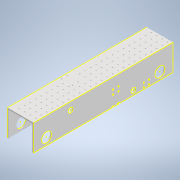
# Autodesk Inventor part: Side Channel
Saved by Autodesk Inventor 2021 (Build 250183000, 183)
## iProperties
Created: 2019-12-09
Part Number: Side Channel
Material: Generic
Document SubType Name: Modeling
Designer: deli
Density: 1 g/cm^3
Appearance: Default
Author: deli
Autodesk Inventor part; units mm, degrees
ref_plane "YZ Plane" through (0, 0, 0) normal (1, 0, 0) x (0, 1, 0)
ref_plane "XZ Plane" through (0, 0, 0) normal (0, 1, 0) x (-1, 0, 0)
ref_plane "XY Plane" through (0, 0, 0) normal (0, 0, 1) x (1, 0, 0)
sketch "Sketch1" plane through (0, 0, 0) normal (0, 0, 1) x (1, 0, 0)
  line L0 (-186.621, 45.7633) -> (-110.421, 45.7633)
  line L1 (-110.421, 45.7633) -> (-110.421, -30.4367)
  line L2 (-110.421, -30.4367) -> (-186.621, -30.4367)
  line L3 (-186.621, -30.4367) -> (-186.621, 45.7633)
  line L4 (-183.446, 42.5883) -> (-113.596, 42.5883)
  line L5 (-113.596, 42.5883) -> (-113.596, -27.2617)
  line L6 (-113.596, -27.2617) -> (-183.446, -27.2617)
  line L7 (-183.446, -27.2617) -> (-183.446, 42.5883)
  point P0 (0, 0)
  dimension "d0" = 76.2
  dimension "d1" = 76.2
  dimension "d2" = 3.175
  dimension "d3" = 3.175
  dimension "d4" = 3.175
  dimension "d5" = 3.175
  constraints: 16 end point, 4 parallel, 2 horizontal, 2 perpendicular
  measures "d0" distance of L1.end L2.end
  measures "d1" distance of L0.end L1.end
  measures "d2" distance between parallel lines of L0 L4
  measures "d3" distance between parallel lines of L1 L5
  measures "d4" distance between parallel lines of L2 L6
  measures "d5" distance between parallel lines of L3 L7
extrude "Extrusion1" add sketch "Sketch1" along normal blind 406.4
sketch "Sketch2" plane through (0, 0, 406.4) normal (0, 0, 1) x (1, 0, 0)
  line L0 (-113.596, 42.5883) -> (-113.596, -27.2617) projected
  line L1 (-183.446, -27.2617) -> (-183.446, 42.5883) projected
  line L2 (-186.621, -30.4367) -> (-110.421, -30.4367) projected
  line L3 (-183.446, -27.2617) -> (-113.596, -27.2617)
  line L4 (-113.596, -27.2617) -> (-113.596, -30.4367)
  line L5 (-113.596, -30.4367) -> (-183.446, -30.4367)
  line L6 (-183.446, -30.4367) -> (-183.446, -27.2617)
  point P0 (0, 0)
  constraints: 8 end point, 2 parallel, 1 horizontal, 1 perpendicular, 1 point on line
extrude "Extrusion2" cut sketch "Sketch2" against normal blind 457.2
sketch "Sketch3" plane through (-110.421, -30.4367, 0) normal (1, 0, 0) x (0, 0, -1)
  circle A0 centre (-368.3, 20.8534) radius 14.5034
  line L0 (-406.4, 0) -> (-406.4, 76.2) projected
  line L1 (0, 0) -> (-406.4, 0) projected
  circle A1 centre (-38.1, 20.8534) radius 14.5034
  line L2 (0, 0) -> (0, 76.2) projected
  point P0 (0, 30.4367)
  dimension "d10" = 29.0068
  dimension "d11" = 38.1
  dimension "d12" = 20.8534
  dimension "d13" = 29.0068
  dimension "d14" = 38.1
  dimension "d15" = 20.8534
  constraints: 2 centre point
  measures "d10" diameter of A0
  measures "d11" distance from line of A0.centre L0
  measures "d12" distance from line of L1 A0.centre
  measures "d13" diameter of A1
  measures "d14" distance from line of L2 A1.centre
  measures "d15" distance from line of L1 A1.centre
extrude "Extrusion3" cut sketch "Sketch3" against normal blind 76.2
sketch "Sketch4" plane through (-186.621, -30.4367, 0) normal (-1, 0, 0) x (0, 0, 1)
  circle A0 centre (115.1699, 12.7) radius 6.9977
  line L0 (0, 76.2) -> (406.4, 76.2) projected
  circle A1 centre (38.1, 20.8534) radius 14.5034 projected
  circle A2 centre (38.1, 20.8534) radius 50.8
  line L1 (0, 0) -> (406.4, 0) projected
  line L2 (88.9, 0) -> (88.9, 76.2)
  circle A3 centre (298.2343, 53.975) radius 6.9977
  circle A4 centre (368.3, 20.8534) radius 2.55 projected
  point P0 (0, 30.4367)
  dimension "d18" = 13.9954
  dimension "d20" = 101.6
  dimension "d21" = 77.5
  dimension "d24" = 13.9954
  dimension "d25" = 22.225
  dimension "d26" = 77.5
  dimension "d31" = 12.7
  constraints: 3 centre point, 2 end point, 2 point on line, 1 coincident, 1 perpendicular
  measures "d18" diameter of A0
  measures "d20" diameter of A2
  measures "d21" distance of A0.centre A2.centre
  measures "d24" diameter of A3
  measures "d25" distance from line of L0 A3.centre
  measures "d26" distance of A3.centre A4.centre
  measures "d31" distance from line of L1 A0.centre
extrude "Extrusion5" cut sketch "Sketch4" against normal blind 127 contours A0 | A3
sketch "Sketch5" plane through (-186.621, 45.7633, 0) normal (0, 1, 0) x (1, 0, 0)
  circle A0 centre (6.225, -254.5181) radius 1.8542
  circle A1 centre (6.225, -238.5181) radius 1.8542
  circle A2 centre (38.225, -238.5181) radius 1.8542
  circle A3 centre (38.225, -254.5181) radius 1.8542
  circle A4 centre (6.225, -254.5181) radius 2.8702 projected
  circle A5 centre (38.225, -254.5181) radius 2.5146 projected
  circle A6 centre (38.225, -238.5181) radius 2.5146 projected
  point P0 (186.621, 0)
  dimension "d36" = 3.7084
  dimension "d37" = 0
  dimension "d38" = 0
  dimension "d39" = 0
  dimension "d40" = 3.7084
  dimension "d41" = 3.7084
  dimension "d42" = 3.7084
  constraints: 4 centre point
  measures "d36" diameter of A1
  measures "d37" distance of A4.centre A0.centre
  measures "d38" distance of A5.centre A3.centre
  measures "d39" distance of A6.centre A2.centre
  measures "d40" diameter of A0
  measures "d41" diameter of A3
  measures "d42" diameter of A2
extrude "Extrusion6" cut sketch "Sketch5" against normal blind 25.4 contours A0 | A1 | A2 | A3
sketch "Sketch6" plane through (-110.421, -30.4367, 0) normal (1, 0, 0) x (0, 0, -1)
  circle A0 centre (-158.8823, 31.875) radius 1.8542
  circle A1 centre (-174.8823, 31.875) radius 1.8542
  circle A2 centre (-174.8823, -0.125) radius 1.8542
  circle A3 centre (-158.8823, -0.125) radius 1.8542
  circle A4 centre (-174.8823, 44.45) radius 1.8542
  circle A5 centre (-158.8823, 44.45) radius 1.8542
  circle A6 centre (-174.8823, -0.125) radius 3.81
  circle A7 centre (-158.8823, -0.125) radius 3.81
  circle A8 centre (-85.09, 17.145) radius 1.8542
  circle A9 centre (-85.09, 5.08) radius 1.8542
  circle A10 centre (-69.85, 5.08) radius 1.8542
  circle A11 centre (-69.85, 17.145) radius 1.8542
  line L0 (0, 0) -> (0, 76.2) projected
  line L1 (0, 0) -> (-406.4, 0) projected
  point P0 (0, 30.4367)
  dimension "d34" = 7.62
  dimension "d35" = 7.62
  dimension "d43" = 3.7084
  dimension "d44" = 3.7084
  dimension "d45" = 3.7084
  dimension "d46" = 3.7084
  dimension "d47" = 3.7084
  dimension "d48" = 3.7084
  dimension "d49" = 11.5316
  dimension "d50" = 15.24
  dimension "d51" = 12.065
  dimension "d52" = 12.065
  dimension "d53" = 15.7292
  dimension "d54" = 69.85
  dimension "d55" = 3.7084
  dimension "d56" = 3.7084
  dimension "d57" = 3.7084
  dimension "d58" = 3.7084
  dimension "d59" = 5.08
  constraints: 12 centre point, 2 coincident
  measures "d34" diameter of A6
  measures "d35" diameter of A7
  measures "d43" diameter of A5
  measures "d44" diameter of A0
  measures "d45" diameter of A1
  measures "d46" diameter of A4
  measures "d47" diameter of A2
  measures "d48" diameter of A3
  measures "d50" distance of A9.centre A10.centre
  measures "d51" distance of A11.centre A10.centre
  measures "d52" distance of A8.centre A9.centre
  measures "d54" distance from line of L0 A11.centre
  measures "d55" diameter of A11
  measures "d56" diameter of A8
  measures "d57" diameter of A9
  measures "d58" diameter of A10
  measures "d59" distance from line of L1 A10.centre
extrude "Extrusion7" cut sketch "Sketch6" against normal blind 25.4
sketch "Sketch7" plane through (-186.621, 45.7633, 0) normal (0, 1, 0) x (1, 0, 0)
  circle A0 centre (20.2, -7.62) radius 1.65
  circle A1 centre (38.225, -254.5181) radius 1.8542 projected
  circle A2 centre (6.225, -238.5181) radius 1.8542 projected
  circle A3 centre (38.225, -238.5181) radius 1.8542 projected
  circle A4 centre (6.225, -254.5181) radius 1.8542 projected
  line L0 (76.2, 0) -> (0, 0) projected
  line L1 (0, 0) -> (0, -406.4) projected
  line L2 (76.2, -406.4) -> (0, -406.4) projected
  line L3 (76.2, 0) -> (76.2, -406.4) projected
  circle A5 centre (36.2, -7.62) radius 1.65
  circle A6 centre (52.2, -7.62) radius 1.65
  circle A7 centre (68.2, -7.62) radius 1.65
  circle A8 centre (20.2, -23.62) radius 1.65
  circle A9 centre (36.2, -23.62) radius 1.65
  circle A10 centre (52.2, -23.62) radius 1.65
  circle A11 centre (68.2, -23.62) radius 1.65
  circle A12 centre (20.2, -39.62) radius 1.65
  circle A13 centre (36.2, -39.62) radius 1.65
  circle A14 centre (52.2, -39.62) radius 1.65
  circle A15 centre (68.2, -39.62) radius 1.65
  circle A16 centre (20.2, -55.62) radius 1.65
  circle A17 centre (36.2, -55.62) radius 1.65
  circle A18 centre (52.2, -55.62) radius 1.65
  circle A19 centre (68.2, -55.62) radius 1.65
  circle A20 centre (20.2, -71.62) radius 1.65
  circle A21 centre (36.2, -71.62) radius 1.65
  circle A22 centre (52.2, -71.62) radius 1.65
  circle A23 centre (68.2, -71.62) radius 1.65
  circle A24 centre (20.2, -87.62) radius 1.65
  circle A25 centre (36.2, -87.62) radius 1.65
  circle A26 centre (52.2, -87.62) radius 1.65
  circle A27 centre (68.2, -87.62) radius 1.65
  circle A28 centre (20.2, -103.62) radius 1.65
  circle A29 centre (36.2, -103.62) radius 1.65
  circle A30 centre (52.2, -103.62) radius 1.65
  circle A31 centre (68.2, -103.62) radius 1.65
  circle A32 centre (20.2, -119.62) radius 1.65
  circle A33 centre (36.2, -119.62) radius 1.65
  circle A34 centre (52.2, -119.62) radius 1.65
  circle A35 centre (68.2, -119.62) radius 1.65
  circle A36 centre (20.2, -135.6199) radius 1.65
  circle A37 centre (36.2, -135.6199) radius 1.65
  circle A38 centre (52.2, -135.6199) radius 1.65
  circle A39 centre (68.2, -135.6199) radius 1.65
  circle A40 centre (20.2, -151.6199) radius 1.65
  circle A41 centre (36.2, -151.6199) radius 1.65
  circle A42 centre (52.2, -151.6199) radius 1.65
  circle A43 centre (68.2, -151.6199) radius 1.65
  circle A44 centre (20.2, -167.6199) radius 1.65
  circle A45 centre (36.2, -167.6199) radius 1.65
  circle A46 centre (52.2, -167.6199) radius 1.65
  circle A47 centre (68.2, -167.6199) radius 1.65
  circle A48 centre (20.2, -183.6199) radius 1.65
  circle A49 centre (36.2, -183.6199) radius 1.65
  circle A50 centre (52.2, -183.6199) radius 1.65
  circle A51 centre (68.2, -183.6199) radius 1.65
  circle A52 centre (20.2, -199.6199) radius 1.65
  circle A53 centre (36.2, -199.6199) radius 1.65
  circle A54 centre (52.2, -199.6199) radius 1.65
  circle A55 centre (68.2, -199.6199) radius 1.65
  circle A56 centre (20.2, -215.6199) radius 1.65
  circle A57 centre (36.2, -215.6199) radius 1.65
  circle A58 centre (52.2, -215.6199) radius 1.65
  circle A59 centre (68.2, -215.6199) radius 1.65
  circle A60 centre (20.2, -231.6199) radius 1.65
  circle A61 centre (36.2, -231.6199) radius 1.65
  circle A62 centre (52.2, -231.6199) radius 1.65
  circle A63 centre (68.2, -231.6199) radius 1.65
  circle A64 centre (20.2, -247.6199) radius 1.65
  circle A65 centre (36.2, -247.6199) radius 1.65
  circle A66 centre (52.2, -247.6199) radius 1.65
  circle A67 centre (68.2, -247.6199) radius 1.65
  circle A68 centre (20.2, -263.6199) radius 1.65
  circle A69 centre (36.2, -263.6199) radius 1.65
  circle A70 centre (52.2, -263.6199) radius 1.65
  circle A71 centre (68.2, -263.6199) radius 1.65
  circle A72 centre (20.2, -279.6199) radius 1.65
  circle A73 centre (36.2, -279.6199) radius 1.65
  circle A74 centre (52.2, -279.6199) radius 1.65
  circle A75 centre (68.2, -279.6199) radius 1.65
  circle A76 centre (20.2, -295.6199) radius 1.65
  circle A77 centre (36.2, -295.6199) radius 1.65
  circle A78 centre (52.2, -295.6199) radius 1.65
  circle A79 centre (68.2, -295.6199) radius 1.65
  circle A80 centre (20.2, -311.6199) radius 1.65
  circle A81 centre (36.2, -311.6199) radius 1.65
  circle A82 centre (52.2, -311.6199) radius 1.65
  circle A83 centre (68.2, -311.6199) radius 1.65
  circle A84 centre (20.2, -327.6199) radius 1.65
  circle A85 centre (36.2, -327.6199) radius 1.65
  circle A86 centre (52.2, -327.6199) radius 1.65
  circle A87 centre (68.2, -327.6199) radius 1.65
  circle A88 centre (20.2, -343.6199) radius 1.65
  circle A89 centre (36.2, -343.6199) radius 1.65
  circle A90 centre (52.2, -343.6199) radius 1.65
  circle A91 centre (68.2, -343.6199) radius 1.65
  circle A92 centre (20.2, -359.6199) radius 1.65
  circle A93 centre (36.2, -359.6199) radius 1.65
  circle A94 centre (52.2, -359.6199) radius 1.65
  circle A95 centre (68.2, -359.6199) radius 1.65
  circle A96 centre (20.2, -375.6198) radius 1.65
  circle A97 centre (36.2, -375.6198) radius 1.65
  circle A98 centre (52.2, -375.6198) radius 1.65
  circle A99 centre (68.2, -375.6198) radius 1.65
  circle A100 centre (20.2, -391.6198) radius 1.65
  circle A101 centre (36.2, -391.6198) radius 1.65
  circle A102 centre (52.2, -391.6198) radius 1.65
  circle A103 centre (68.2, -391.6198) radius 1.65
  circle A104 centre (84.2, -71.62) radius 1.65 projected
  circle A105 centre (84.2, -87.62) radius 1.65 projected
  point P0 (186.621, 0)
  dimension "d60" = 3.3
  dimension "d63" = 16
  dimension "d66" = 16
  dimension "d69" = 8
  dimension "d70" = 383.9998
  dimension "d71" = 7.62
  constraints: 100 centre point, 1 horizontal, 1 vertical, 198 other
  measures "d60" diameter of A0
  measures "d63" distance of A0.centre A5.centre
  measures "d66" distance of A0.centre A8.centre
  measures "d69" distance from line of L3 A7.centre
  measures "d70" distance of A102.centre A6.centre
  measures "d71" distance from line of A6.centre L0
extrude "Extrusion8" cut sketch "Sketch7" against normal blind 25.4 contours A0 | A5 | A6 | A7 | A8 | A9 | A10 | A11 | A12 | A13 | A14 | A15 | A16 | A17 | A18 | A19 | A20 | A21 | A22 | A23 | A24 | A25 | A26 | A27 | A28 | A29 | A30 | A31 | A32 | A33 | A34 | A35 | A36 | A37 | A38 | A39 | A40 | A41 | A42 | A43 | A44 | A45 | A46 | A47 | A48 | A49 | A50 | A51 | A52 | A53 | A54 | A55 | A56 | A57 | A58 | A59 | A62 | A63 | A66 | A67 | A68 | A69 | A70 | A71 | A72 | A73 | A74 | A75 | A76 | A77 | A78 | A79 | A80 | A81 | A82 | A83 | A84 | A85 | A86 | A87 | A88 | A89 | A90 | A91 | A92 | A93 | A94 | A95 | A96 | A97 | A98 | A99 | A100 | A101 | A102 | A103
sketch "Sketch10" plane through (-110.421, -30.4367, 0) normal (1, 0, 0) x (0, 0, -1)
  arc A0 (-155.0743, 0) -> (-162.6902, 0) centre (-158.8823, -0.125) ccw projected
  line L0 (0, 0) -> (-155.0743, 0) projected
  line L1 (0, 0) -> (0, 76.2) projected
  line L2 (0, 76.2) -> (-406.4, 76.2) projected
  line L3 (-406.4, 0) -> (-406.4, 76.2) projected
  line L4 (-178.6902, 0) -> (-406.4, 0) projected
  arc A1 (-171.0743, 0) -> (-178.6902, 0) centre (-174.8823, -0.125) ccw projected
  line L5 (-162.6902, 0) -> (-171.0743, 0) projected
  circle A2 centre (-69.85, 5.08) radius 1.8542 projected
  circle A3 centre (-174.8823, 31.875) radius 1.8542 projected
  circle A4 centre (-174.8823, 44.45) radius 1.8542 projected
  circle A5 centre (-85.09, 5.08) radius 1.8542 projected
  circle A6 centre (-69.85, 17.145) radius 1.8542 projected
  circle A7 centre (-158.8823, 31.875) radius 1.8542 projected
  circle A8 centre (-158.8823, 44.45) radius 1.8542 projected
  circle A9 centre (-85.09, 17.145) radius 1.8542 projected
  circle A10 centre (-298.2343, 53.975) radius 6.9977 projected
  circle A11 centre (-115.1699, 12.7) radius 6.9977 projected
  circle A12 centre (-38.1, 20.8534) radius 14.5034 projected
  circle A13 centre (-368.3, 20.8534) radius 14.5034 projected
  point P0 (0, 30.4367)
sketch "Sketch11" plane through (-186.621, -30.4367, 0) normal (-1, 0, 0) x (0, 0, 1)
  circle A0 centre (298.2343, 53.975) radius 6.9977 projected
  circle A1 centre (115.1699, 12.7) radius 6.9977 projected
  circle A2 centre (38.1, 20.8534) radius 14.5034 projected
  circle A3 centre (368.3, 20.8534) radius 14.5034 projected
  line L0 (0, 76.2) -> (0, 0) projected
  line L1 (0, 0) -> (406.4, 0) projected
  line L2 (406.4, 76.2) -> (406.4, 0) projected
  line L3 (0, 76.2) -> (406.4, 76.2) projected
  point P0 (0, 30.4367)
equation "\"d3\" = d2"
equation "\"d4\" = d2"
equation "\"d5\" = d2"
equation "\"d13\" = d10"
equation "\"d14\" = d11"
equation "\"d15\" = d12"
equation "\"d25\" = d19"
equation "\"d26\" = d21"
equation "\"d40\" = d36"
equation "\"d41\" = d36"
equation "\"d42\" = d36"
equation "\"d44\" = d43"
equation "\"d45\" = d44"
equation "\"d46\" = d43"
equation "\"d47\" = d45"
equation "\"d48\" = d44"
equation "\"d19\" = 22.225"
body "Solid1"
